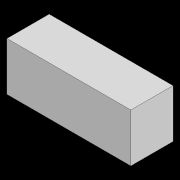
# Autodesk Inventor part: Battery Mockup
Saved by Autodesk Inventor 2021 (Build 250183000, 183)
## iProperties
Created: 2021-03-28
Part Number: Battery Mockup
Material: Generic
Document SubType Name: Modeling
Designer: Esketitttttt
Density: 1.9154 g/cm^3
Appearance: Default
Mass: 693 g
Surface Area: 336.741 cm^2
Volume: 361.804 cm^3
Author: Esketitttttt
Autodesk Inventor part; units mm, degrees
ref_plane "YZ Plane" through (0, 0, 0) normal (1, 0, 0) x (0, 1, 0)
ref_plane "XZ Plane" through (0, 0, 0) normal (0, 1, 0) x (-1, 0, 0)
ref_plane "XY Plane" through (0, 0, 0) normal (0, 0, 1) x (1, 0, 0)
sketch "Sketch1" plane through (0, 0, 0) normal (0, 1, 0) x (-1, 0, 0)
  line L0 (0, 0) -> (139.54, 0)
  line L1 (139.54, 0) -> (139.54, -47.54)
  line L2 (139.54, -47.54) -> (0, -47.54)
  line L3 (0, -47.54) -> (0, 0)
  dimension "d0" = 139.54
  dimension "d1" = 47.54
  constraints: 8 end point, 2 parallel, 1 horizontal, 1 perpendicular
  measures "d0" distance of L1.end L2.end
  measures "d1" distance of L0.end L1.end
extrude "Extrusion1" add sketch "Sketch1" along normal blind 54.54
body "Solid1"
